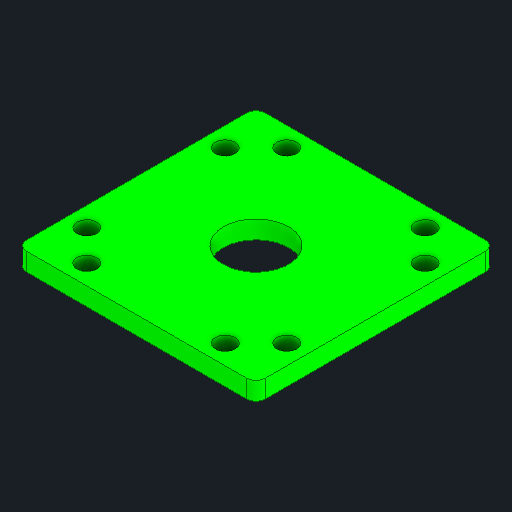
# Autodesk Inventor part: Top Mount (SM05)
Saved by Autodesk Inventor 2023.4 (Build 274418000, 418)
## iProperties
Created: 2022-07-25
Part Number: Top Mount (SM05)
Material: Generic
Document SubType Name: Modeling
Designer: xSibe
Density: 1 g/cm^3
Appearance: Plastic Green
Author: xSibe
Autodesk Inventor part; units mm, degrees
ref_plane "YZ Plane" through (0, 0, 0) normal (1, 0, 0) x (0, 1, 0)
ref_plane "XZ Plane" through (0, 0, 0) normal (0, 1, 0) x (-1, 0, 0)
ref_plane "XY Plane" through (0, 0, 0) normal (0, 0, 1) x (1, 0, 0)
sketch "Sketch1" plane through (0, 0, 0) normal (0, 1, 0) x (-1, 0, 0)
  circle A0 centre (-20.8, 14.4) radius 6.7838
  circle A1 centre (-42.7, -7.5) radius 1.875 projected
  circle A2 centre (1.1, 36.3) radius 1.875 projected
  circle A3 centre (1.1, -7.5) radius 1.875 projected
  circle A4 centre (-42.7, 36.3) radius 1.875 projected
  circle A5 centre (-6.4, 35.2) radius 2.0734 projected
  circle A6 centre (-35.2, -6.4) radius 2.0734 projected
  circle A7 centre (-6.4, -6.4) radius 2.0734 projected
  circle A8 centre (0, 0) radius 2.0734 projected
  line L0 (-37.85, 31.45) -> (-37.85, -2.65) projected
  line L1 (-3.75, 31.45) -> (-37.85, 31.45) projected
  line L2 (-3.75, -2.65) -> (-3.75, 31.45) projected
  line L3 (-37.85, -2.65) -> (-3.75, -2.65) projected
  circle A9 centre (0, 28.8) radius 2.0734 projected
  circle A10 centre (-35.2, 35.2) radius 2.0734 projected
  circle A11 centre (-41.6, 0) radius 2.0734 projected
  circle A12 centre (-41.6, 28.8) radius 2.0734 projected
  line L4 (-43.7, 39.275) -> (2.1, 39.275) projected
  arc A13 (-43.7, 39.275) -> (-45.675, 37.3) centre (-43.7, 37.3) ccw projected
  line L5 (-45.675, -8.5) -> (-45.675, 37.3) projected
  arc A14 (-45.675, -8.5) -> (-43.7, -10.475) centre (-43.7, -8.5) ccw projected
  line L6 (2.1, -10.475) -> (-43.7, -10.475) projected
  arc A15 (2.1, -10.475) -> (4.075, -8.5) centre (2.1, -8.5) ccw projected
  line L7 (4.075, 37.3) -> (4.075, -8.5) projected
  arc A16 (4.075, 37.3) -> (2.1, 39.275) centre (2.1, 37.3) ccw projected
  line L8 (-3.75, 14.4) -> (-37.85, 14.4)
  dimension "d36" = 13.5675
  constraints: 3 midpoint, 2 end point, 1 centre point
  measures "d36" diameter of A0
extrude "Extrusion1" add sketch "Sketch1" along normal blind 3.75 contours L8 L2 L3 L0 A0 | A0 L8 L0 L1 L2 | A1 | A2 | A3 | A4 | L4 A16 L7 A15 L6 A14 L5 A13
body "Solid1"
